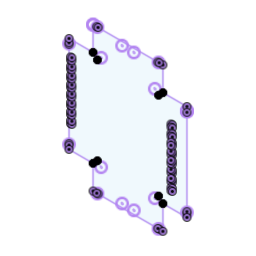
pencil case clasp 2 v8 (Autodesk Fusion 360 design; units mm, degrees)
Autodesk Fusion 360 part; units mm, degrees
sketch "end" plane through (0, 0, 0) normal (0, 1, 0) x (1, 0, 0)
  line L0 (0, 0) -> (10, 0)
  line L1 (10, 0) -> (10, 6)
  line L2 (10, 6) -> (0, 6)
  line L3 (0, 6) -> (0, 0)
  line L4 (0, 0) -> (-10, 0)
  line L5 (-10, 0) -> (-10, 6)
  line L6 (-10, 6) -> (0, 6)
  line L7 (0, 6) -> (0, 0)
  line L8 (0, 3) -> (10, 3) construction
  line L9 (0, 1.2) -> (2, 3)
  line L10 (2, 3) -> (0, 4.8)
  dimension "d1" = 10
  dimension "d2" = 6
  dimension "d3" = 10
  dimension "d4" = 6
  dimension "d5" = 1.2
  dimension "d6" = 1.2
  dimension "d99" = 2
  constraint horizontal L0
  constraint vertical L1
  constraint horizontal L2
  constraint vertical L3
  constraint coincident L0.start L3.end
  constraint horizontal L4
  constraint vertical L5
  constraint horizontal L6
  constraint vertical L7
  constraint midpoint L7 L8.start
  constraint midpoint L1 L8.end
  constraint coincident L3 L9.start
  constraint coincident L3 L10.end
  constraint coincident L8 L9.end
  measures "d1" distance of L0.start L0.end
  measures "d2" distance of L0.start L2.end
  measures "d3" distance of L0.start L4.end
  measures "d4" distance of L0.start L2.end
  measures "d5" distance of L0 L9.start
  measures "d6" distance of L2 L10.end
  measures "d99" distance of L7 L9.end
extrude "Extrude1" add sketch "end" along normal blind 80 contours L0 L1 L2 L3 L7 L9 L10 makes body 1
extrude "Extrude2" add sketch "end" along normal blind 80 separate body contours L3 L4 L5 L6 L7 | L3 L7 L9 L10 makes body 2
sketch "latch" plane through (0, 0, -6) normal (0, 0, -1) x (-1, 0, 0)
  line L0 (-10, 0) -> (0, 0)
  line L1 (0, 0) -> (0, 80)
  line L2 (0, 80) -> (-10, 80)
  line L3 (-10, 80) -> (-10, 0)
  line L4 (0, 0) -> (10, 0)
  line L5 (10, 0) -> (10, 80)
  line L6 (10, 80) -> (0, 80)
  line L7 (0, 80) -> (0, 0)
  line L8 (-10, 0) -> (0, 0)
  line L9 (5, 80) -> (5, 0) construction
  line L10 (10, 66) -> (5, 66)
  line L11 (5, 74) -> (0, 74)
  line L12 (5, 66) -> (5, 74)
  line L13 (5, 66) -> (4.5, 66)
  line L14 (4.5, 66) -> (4.5, 74)
  line L15 (10, 6) -> (-10, 6)
  line L16 (-10, 6) -> (-10, 12)
  line L17 (-10, 12) -> (10, 12)
  line L18 (10, 12) -> (10, 6)
  dimension "d100" = 6
  dimension "d101" = 8
  dimension "d102" = 0.5
  dimension "d116" = 20
  dimension "d117" = 6
  dimension "d118" = 6
  constraint midpoint L6 L9.start
  constraint midpoint L4 L9.end
  constraint coincident L5 L10.start
  constraint coincident L9 L10.end
  constraint perpendicular L9 L10
  constraint coincident L9 L11.start
  constraint coincident L1 L11.end
  constraint perpendicular L1 L11
  constraint perpendicular L9 L13
  constraint coincident L11 L14.end
  constraint perpendicular L11 L14
  constraint horizontal L15
  constraint vertical L16
  constraint horizontal L17
  constraint vertical L18
  constraint coincident L5 L15.start
  measures "d100" distance of L6 L11
  measures "d101" distance of L10 L11
  measures "d102" distance of L10.end L13.end
  measures "d116" distance of L15.start L15.end
  measures "d117" distance of L15.start L17.end
  measures "d118" distance of L4 L15
extrude "Extrude3" cut sketch "latch" against normal blind 6 contours L1 L5 L6 L7 L10 L11 L12 | L11 L12 L13 L14 bodies 2
extrude "Extrude4" add sketch "latch" against normal blind 6 contours L1 L5 L6 L7 L10 L11 L12 bodies 1
extrude "Extrude5" cut 1 faces at (0, 76, -3.6) along direction (1, 0, 0) blind 5 on bodies 2 bodies 2
extrude "Extrude6" add 1 faces at (0, 76, -3.6) along direction (1, 0, 0) blind 4 on bodies 1 bodies 1
chamfer "Chamfer5" distance 2 angle 45 2 edges at (-5, 66, -3) (-4.5, 74, -3) on bodies 1 2
fillet "Fillet8" radius 2 1 edges at (-10, 66, -3) on bodies 1
fillet "Fillet9" radius 2 1 edges at (-10, 66, -3) on bodies 2
fillet "Fillet10" radius 3 2 edges at (-10, 80, -3) (10, 80, -3) on bodies 1
extrude "Extrude16" add sketch "latch" along normal blind 6 contours L1 L3 L7 L15 L16 L17 | L1 L5 L7 L15 L17 L18 bodies 2
fillet "Fillet11" radius 3 4 edges at (10, 12, -9) (10, 6, -9) (-10, 6, -9) (-10, 12, -9) on bodies 2
fillet "Fillet12" radius 2 4 edges at (-10, 9, -12) (0, 12, -12) (10, 9, -12) (0, 6, -12) on bodies 2
sketch "detent" plane through (0, 0, 0) normal (0, 0, 1) x (1, 0, 0)
  arc A0 (-8, 66) -> (-10, 64) centre (-8, 64) ccw
  line L0 (-10, 64) -> (-10, 0)
  line L1 (-10, 0) -> (0, 0)
  line L2 (0, 0) -> (0, 74)
  line L3 (0, 74) -> (-2.5, 74)
  line L4 (-2.5, 74) -> (-4.5, 72)
  line L5 (-4.5, 72) -> (-4.5, 66)
  line L6 (-4.5, 66) -> (-8, 66)
  line L7 (2, 74) -> (0, 74)
  line L8 (0, 74) -> (0, 0)
  line L9 (0, 0) -> (2, 0)
  line L10 (2, 0) -> (2, 74)
  arc A1 (7, 6) -> (7, 12) centre (7, 9) ccw
  line L11 (7, 12) -> (0, 12)
  line L12 (0, 12) -> (0, 6)
  line L13 (0, 6) -> (7, 6)
  circle A2 centre (2, 17) radius 2
  dimension "d133" = 4
  dimension "d134" = 5
  constraint coincident L10 A2.centre
  measures "d133" diameter of A2
  measures "d134" distance of L11 A2.centre
extrude "Extrude17" add sketch "detent" against normal blind 6 contours L10 A2 | L10 A2 bodies 1
extrude "Extrude18" cut sketch "detent" against normal blind 6 contours L10 A2 | L10 A2 bodies 2
copy_body "CopyPasteBodies1" bodies 2 makes body 3
move_body "Move1" bodies 3 to x (-1, 0, 0) y (0, -1, 0) z (0, 0, 1) at (0, 0, 0)
combine "Combine1" operation add target body 1 tool bodies 3
extrude "Extrude9" cut 1 faces at (0.6667, 0, -3) along direction (0, -1, 0) blind 10 on bodies 1 bodies 1
sketch "pins" plane through (0, 0, 0) normal (0, 0, 1) x (1, 0, 0)
  line L0 (10, -64) -> (10, 77)
  line L1 (7, 80) -> (-7, 80)
  line L2 (0, 74) -> (0, -74)
  line L3 (0, 0) -> (18.7462, 0) construction
  line L4 (3.5, 3) -> (6.5, 3)
  line L5 (6.5, 3) -> (6.5, -3)
  line L6 (6.5, -3) -> (3.5, -3)
  line L7 (3.5, -3) -> (3.5, 3)
  line L8 (3.5, 3) -> (6.5, -3) construction
  line L9 (6.5, 3) -> (3.5, -3) construction
  line L10 (6.5, -75) -> (3.5, -75)
  line L11 (3.5, -75) -> (3.5, -69)
  line L12 (3.5, -69) -> (6.5, -69)
  line L13 (6.5, -69) -> (6.5, -75)
  line L14 (6.5, -57) -> (3.5, -57)
  line L15 (3.5, -57) -> (3.5, -51)
  line L16 (3.5, -51) -> (6.5, -51)
  line L17 (6.5, -51) -> (6.5, -57)
  line L18 (6.5, -39) -> (3.5, -39)
  line L19 (3.5, -39) -> (3.5, -33)
  line L20 (3.5, -33) -> (6.5, -33)
  line L21 (6.5, -33) -> (6.5, -39)
  line L22 (6.5, -21) -> (3.5, -21)
  line L23 (3.5, -21) -> (3.5, -15)
  line L24 (3.5, -15) -> (6.5, -15)
  line L25 (6.5, -15) -> (6.5, -21)
  line L26 (6.5, 15) -> (3.5, 15)
  line L27 (3.5, 15) -> (3.5, 21)
  line L28 (3.5, 21) -> (6.5, 21)
  line L29 (6.5, 21) -> (6.5, 15)
  line L30 (6.5, 33) -> (3.5, 33)
  line L31 (3.5, 33) -> (3.5, 39)
  line L32 (3.5, 39) -> (6.5, 39)
  line L33 (6.5, 39) -> (6.5, 33)
  line L34 (6.5, 51) -> (3.5, 51)
  line L35 (3.5, 51) -> (3.5, 57)
  line L36 (3.5, 57) -> (6.5, 57)
  line L37 (6.5, 57) -> (6.5, 51)
  line L38 (6.5, 69) -> (3.5, 69)
  line L39 (3.5, 69) -> (3.5, 75)
  line L40 (3.5, 75) -> (6.5, 75)
  line L41 (6.5, 75) -> (6.5, 69)
  line L42 (9, 80) -> (7, 80)
  line L43 (3.4, -68.9) -> (6.6, -68.9)
  line L44 (6.6, -68.9) -> (6.6, -75.1)
  line L45 (6.6, -75.1) -> (3.4, -75.1)
  line L46 (3.4, -75.1) -> (3.4, -68.9)
  line L47 (3.4, -50.9) -> (6.6, -50.9)
  line L48 (6.6, -50.9) -> (6.6, -57.1)
  line L49 (6.6, -57.1) -> (3.4, -57.1)
  line L50 (3.4, -57.1) -> (3.4, -50.9)
  line L51 (3.4, -32.9) -> (6.6, -32.9)
  line L52 (6.6, -32.9) -> (6.6, -39.1)
  line L53 (6.6, -39.1) -> (3.4, -39.1)
  line L54 (3.4, -39.1) -> (3.4, -32.9)
  line L55 (3.4, -14.9) -> (6.6, -14.9)
  line L56 (6.6, -14.9) -> (6.6, -21.1)
  line L57 (6.6, -21.1) -> (3.4, -21.1)
  line L58 (3.4, -21.1) -> (3.4, -14.9)
  line L59 (3.4, 3.1) -> (6.6, 3.1)
  line L60 (6.6, 3.1) -> (6.6, -3.1)
  line L61 (6.6, -3.1) -> (3.4, -3.1)
  line L62 (3.4, -3.1) -> (3.4, 3.1)
  line L63 (3.4, 21.1) -> (6.6, 21.1)
  line L64 (6.6, 21.1) -> (6.6, 14.9)
  line L65 (6.6, 14.9) -> (3.4, 14.9)
  line L66 (3.4, 14.9) -> (3.4, 21.1)
  line L67 (3.4, 39.1) -> (6.6, 39.1)
  line L68 (6.6, 39.1) -> (6.6, 32.9)
  line L69 (6.6, 32.9) -> (3.4, 32.9)
  line L70 (3.4, 32.9) -> (3.4, 39.1)
  line L71 (3.4, 57.1) -> (6.6, 57.1)
  line L72 (6.6, 57.1) -> (6.6, 50.9)
  line L73 (6.6, 50.9) -> (3.4, 50.9)
  line L74 (3.4, 50.9) -> (3.4, 57.1)
  line L75 (3.4, 75.1) -> (6.6, 75.1)
  line L76 (6.6, 75.1) -> (6.6, 68.9)
  line L77 (6.6, 68.9) -> (3.4, 68.9)
  line L78 (3.4, 68.9) -> (3.4, 75.1)
  arc A0 (10, 77) -> (7, 80) centre (7, 77) ccw
  arc A1 (-7, 80) -> (-10, 77) centre (-7, 77) ccw
  line L79 (-10, 77) -> (-10, 68)
  arc A2 (-10, 68) -> (-8, 66) centre (-8, 68) ccw
  line L80 (-5, 74) -> (0, 74)
  line L81 (0, -74) -> (2.5, -74)
  line L82 (4.5, -72) -> (4.5, -66)
  line L83 (4.5, -66) -> (8, -66)
  arc A3 (8, -66) -> (10, -64) centre (8, -64) ccw
  line L84 (10, -64) -> (0, -64)
  line L85 (0, 74) -> (0, 80)
  line L86 (-7, 66) -> (-5, 68)
  line L87 (-5, 68) -> (-5, 74)
  line L88 (2.5, -74) -> (4.5, -72)
  line L89 (-8, 66) -> (-7, 66)
  point P0 (5, 0)
  dimension "d56" = 3
  dimension "d57" = 6
  dimension "d60" = 0
  dimension "d61" = 18
  dimension "d65" = -0.1
  dimension "d66" = -0.1
  dimension "d67" = -0.1
  dimension "d68" = -0.1
  dimension "d69" = -0.1
  dimension "d70" = -0.1
  dimension "d71" = -0.1
  dimension "d72" = -0.1
  dimension "d73" = -0.1
  dimension "d125" = 5
  constraint coincident L3.start origin
  constraint perpendicular L2 L3
  constraint horizontal L4
  constraint perpendicular L4 L5
  constraint parallel L4 L6
  constraint parallel L5 L7
  constraint coincident L8 P0
  constraint coincident L9 P0
  constraint coincident L3 P0
  constraint coincident L1.start L42.end
  constraint coincident L0.start A3.end
  constraint coincident L2 L84.end
  constraint perpendicular L2 L84
  constraint coincident L2.start L80.end
  constraint midpoint L1 L85.end
  measures "d56" distance of L5.end L6.end
  measures "d57" distance of L4.end L5.end
  measures "d125" distance of L0 P0
extrude "Extrude13" add sketch "pins" along normal blind 2 separate body contours L0 L1 L2 A0 L84 L85 makes body 4
extrude "Extrude14" add sketch "pins" along normal blind 3.5 contours L4 L5 L6 L7 | L14 L15 L16 L17 | L18 L19 L20 L21 | L22 L23 L24 L25 | L26 L27 L28 L29 | L30 L31 L32 L33 | L34 L35 L36 L37 | L38 L39 L40 L41 bodies 1
chamfer "Chamfer4" distance 1 angle 45 32 edges at (5, -57.1, 2) (3.4, -54, 2) (5, -50.9, 2) (6.6, -54, 2) (5, -39.1, 2) (3.4, -36, 2) (5, -32.9, 2) (6.6, -36, 2) (5, -21.1, 2) (3.4, -18, 2) (5, -14.9, 2) (6.6, -18, 2) (5, -3.1, 2) (3.4, 0, 2) (6.6, 0, 2) (5, 3.1, 2) (5, 14.9, 2) (3.4, 18, 2) (6.6, 18, 2) (5, 21.1, 2) (5, 32.9, 2) (3.4, 36, 2) (6.6, 36, 2) (5, 39.1, 2) (5, 50.9, 2) (6.6, 54, 2) (3.4, 54, 2) (5, 57.1, 2) (5, 68.9, 2) (6.6, 72, 2) (3.4, 72, 2) (5, 75.1, 2) tangent chain off on bodies 4
fillet "Fillet4" radius 1 1 faces at (5.8667, -62.0333, 2) on bodies 4
fillet "Fillet5" radius 1 10 edges at (0, 80, -6) (-9.1213, 79.1213, -6) (-10, 72.5, -6) (-9.4142, 66.5858, -6) (-7.5, 66, -6) (9.1213, 79.1213, -6) (10, 34, -6) (10, -36.5, -6) (9.4142, -65.4142, -6) (6.25, -66, -6) on bodies 1
fillet "Fillet6" radius 1 2 edges at (-2, -12.5, -3) (-2, -46.5, -3) on bodies 1
sketch "fabric layout" plane through (0, 0, 0) normal (0, 0, 1) x (1, 0, 0)
  line L0 (3.4, 75.1) -> (6.6, 75.1)
  line L1 (3.4, 57.1) -> (6.6, 57.1)
  line L2 (3.4, 39.1) -> (6.6, 39.1)
  line L3 (3.4, 21.1) -> (6.6, 21.1)
  line L4 (3.4, 3.1) -> (6.6, 3.1)
  line L5 (3.4, -14.9) -> (6.6, -14.9)
  line L6 (3.4, -32.9) -> (6.6, -32.9)
  line L7 (3.4, -50.9) -> (6.6, -50.9)
  line L8 (3.4, -39.1) -> (3.4, -32.9)
  line L9 (6.6, -39.1) -> (3.4, -39.1)
  line L10 (3.4, 68.9) -> (3.4, 75.1)
  line L11 (6.6, 68.9) -> (3.4, 68.9)
  line L12 (3.4, -57.1) -> (3.4, -50.9)
  line L13 (6.6, -57.1) -> (3.4, -57.1)
  line L14 (3.4, 50.9) -> (3.4, 57.1)
  line L15 (6.6, 50.9) -> (3.4, 50.9)
  line L16 (3.4, 32.9) -> (3.4, 39.1)
  line L17 (6.6, 32.9) -> (3.4, 32.9)
  line L18 (3.4, -3.1) -> (3.4, 3.1)
  line L19 (6.6, -3.1) -> (3.4, -3.1)
  line L20 (3.4, 14.9) -> (3.4, 21.1)
  line L21 (6.6, 14.9) -> (3.4, 14.9)
  line L22 (3.4, -21.1) -> (3.4, -14.9)
  line L23 (6.6, -21.1) -> (3.4, -21.1)
  line L24 (0, -64) -> (0, 80)
  line L25 (7, 80) -> (0, 80)
  line L26 (0, 0) -> (0, 100) construction
  line L27 (0, 100) -> (30, 100) construction
  line L28 (30, 100) -> (90, 100) construction
  line L29 (90, 100) -> (120, 100) construction
  line L30 (0, 0) -> (0, 165)
  line L31 (0, 165) -> (120, 165)
  circle A0 centre (0, 100) radius 1.5
  line L32 (120, 165) -> (120, 2.0082) construction
  line L33 (236.6, -50.9) -> (233.4, -50.9)
  line L34 (236.6, -57.1) -> (236.6, -50.9)
  line L35 (150, 100) -> (120, 100) construction
  line L36 (233.4, -21.1) -> (236.6, -21.1)
  line L37 (236.6, -14.9) -> (233.4, -14.9)
  line L38 (236.6, -32.9) -> (233.4, -32.9)
  line L39 (233.4, -3.1) -> (236.6, -3.1)
  line L40 (233.4, -57.1) -> (236.6, -57.1)
  line L41 (233.4, -50.9) -> (233.4, -57.1)
  line L42 (240, 165) -> (120, 165)
  line L43 (236.6, -21.1) -> (236.6, -14.9)
  line L44 (236.6, 3.1) -> (233.4, 3.1)
  line L45 (236.6, -3.1) -> (236.6, 3.1)
  line L46 (233.4, -39.1) -> (236.6, -39.1)
  line L47 (233.4, 3.1) -> (233.4, -3.1)
  line L48 (233.4, 21.1) -> (233.4, 14.9)
  line L49 (236.6, 21.1) -> (233.4, 21.1)
  line L50 (233.4, 32.9) -> (236.6, 32.9)
  line L51 (236.6, 57.1) -> (233.4, 57.1)
  line L52 (233.4, 50.9) -> (236.6, 50.9)
  line L53 (233.4, 57.1) -> (233.4, 50.9)
  line L54 (240, 100) -> (210, 100) construction
  line L55 (210, 100) -> (150, 100) construction
  line L56 (236.6, 50.9) -> (236.6, 57.1)
  line L57 (236.6, 39.1) -> (233.4, 39.1)
  line L58 (240, 0) -> (240, 100) construction
  line L59 (233.4, 39.1) -> (233.4, 32.9)
  line L60 (236.6, -39.1) -> (236.6, -32.9)
  line L61 (236.6, 32.9) -> (236.6, 39.1)
  line L62 (233.4, -32.9) -> (233.4, -39.1)
  line L63 (233.4, -14.9) -> (233.4, -21.1)
  line L64 (236.6, 14.9) -> (236.6, 21.1)
  line L65 (233.4, 14.9) -> (236.6, 14.9)
  line L66 (240, 165) -> (270, 165)
  line L67 (0, 0) -> (393.973, 0) construction
  line L68 (270, 165) -> (270, 0)
  arc A1 (10, 77) -> (7, 80) centre (7, 77) ccw
  line L69 (10, -64) -> (10, 77)
  line L70 (6.6, 75.1) -> (6.6, 68.9)
  line L71 (6.6, 57.1) -> (6.6, 50.9)
  line L72 (6.6, 39.1) -> (6.6, 32.9)
  line L73 (6.6, 21.1) -> (6.6, 14.9)
  line L74 (6.6, 3.1) -> (6.6, -3.1)
  line L75 (6.6, -14.9) -> (6.6, -21.1)
  line L76 (6.6, -32.9) -> (6.6, -39.1)
  line L77 (6.6, -50.9) -> (6.6, -57.1)
  line L78 (10, -64) -> (0, -64)
  line L79 (0, 100) -> (65, 100)
  line L80 (65, 100) -> (65, 165)
  line L81 (270, 100) -> (205, 100)
  line L82 (205, 100) -> (205, 165)
  line L83 (140, 165) -> (205, 100) construction
  line L84 (130, 165) -> (65, 100) construction
  line L85 (130, 165) -> (181.9186, 165) construction
  circle A2 centre (65, 100) radius 1.5
  circle A3 centre (205, 100) radius 1.5
  line L86 (270, 110) -> (268.1505, 110)
  line L87 (268.1505, 110) -> (215, 110)
  line L88 (215, 110) -> (215, 165)
  line L89 (55, 165) -> (55, 110)
  line L90 (55, 110) -> (0, 110)
  line L91 (55, 110) -> (65, 100)
  line L92 (205, 100) -> (215, 110)
  circle A4 centre (121.5147, 156.5147) radius 1.5
  circle A5 centre (73.4853, 108.4853) radius 1.5
  circle A6 centre (196.5147, 108.4853) radius 1.5
  circle A7 centre (148.4853, 156.5147) radius 1.5
  line L93 (0, 0) -> (0, -100) construction
  line L94 (0, 0) -> (0, -165)
  line L95 (55, -110) -> (0, -110)
  line L96 (0, -100) -> (65, -100)
  line L97 (55, -110) -> (65, -100)
  line L98 (65, -100) -> (130, -165)
  line L99 (55, -165) -> (55, -110)
  line L100 (0, -165) -> (120, -165)
  line L101 (130, -165) -> (181.9186, -165) construction
  line L102 (240, -165) -> (120, -165)
  line L103 (205, -100) -> (140, -165)
  line L104 (205, -100) -> (215, -110)
  line L105 (240, -100) -> (210, -100) construction
  line L106 (270, -100) -> (205, -100)
  line L107 (268.1505, -110) -> (215, -110)
  line L108 (215, -110) -> (215, -165)
  line L109 (270, -165) -> (270, 0)
  line L110 (240, -165) -> (270, -165)
  circle A8 centre (121.5147, -156.5147) radius 1.5
  circle A9 centre (73.4853, -108.4853) radius 1.5
  circle A10 centre (196.5147, -108.4853) radius 1.5
  circle A11 centre (270, 100) radius 1.5
  circle A12 centre (0, -100) radius 1.5
  circle A13 centre (65, -100) radius 1.5
  circle A14 centre (130, -165) radius 1.5
  circle A15 centre (121.5147, -156.5147) radius 1.5
  circle A16 centre (73.4853, -108.4853) radius 1.5
  circle A17 centre (196.5147, -108.4853) radius 1.5
  circle A18 centre (148.4853, -156.5147) radius 1.5
  circle A19 centre (205, -100) radius 1.5
  circle A20 centre (270, -100) radius 1.5
  line L111 (233.4, -68.9) -> (236.6, -68.9)
  line L112 (233.4, -75.1) -> (233.4, -68.9)
  line L113 (236.6, -68.9) -> (236.6, -75.1)
  line L114 (236.6, -75.1) -> (233.4, -75.1)
  line L115 (268.1505, -110) -> (215, -110)
  line L116 (270, -110) -> (268.1505, -110)
  circle A21 centre (65, 165) radius 1.5
  circle A22 centre (205, 165) radius 1.5
  line L117 (65, -100) -> (65, -165)
  line L118 (205, -100) -> (205, -165)
  circle A23 centre (205, -165) radius 1.5
  circle A24 centre (65, -165) radius 1.5
  point P0 (7, 80)
  point P1 (233, 80)
  point P2 (240, 0)
  point P3 (120, 2.0082)
  point P4 (148.4853, -156.5147)
  dimension "d85" = 100
  dimension "d86" = 30
  dimension "d87" = 60
  dimension "d88" = 30
  dimension "d89" = 20
  dimension "d90" = 65
  dimension "d91" = 3
  dimension "d92" = 120
  dimension "d93" = 30
  dimension "d143" = 65
  dimension "d144" = 65
  dimension "d145" = 315
  dimension "d146" = 135
  dimension "d147" = 30
  dimension "d148" = 3
  dimension "d149" = 3
  dimension "d150" = 10
  dimension "d151" = 10
  dimension "d152" = 10
  dimension "d153" = 10
  dimension "d154" = 3
  dimension "d155" = 3
  dimension "d156" = 3
  dimension "d157" = 3
  dimension "d158" = 12
  dimension "d159" = 12
  dimension "d160" = 12
  dimension "d161" = 12
  dimension "d162" = 65
  dimension "d165" = 3
  dimension "d166" = 3
  dimension "d167" = 3
  constraint coincident L26.start L30.start
  constraint perpendicular L4 L26
  constraint perpendicular L24 L27
  constraint parallel L27 L28
  constraint parallel L28 L29
  constraint perpendicular L27 L30
  constraint perpendicular L26 L31
  constraint coincident L26.end L27.start
  constraint perpendicular L31 L32
  constraint symmetric L26.start L32 P2
  constraint symmetric L1.end L32 L51.end
  constraint symmetric L15.start L32 L52.start
  constraint symmetric L1.start L32 L51.start
  constraint symmetric L2.end L32 L57.end
  constraint symmetric L17.start L32 L50.start
  constraint symmetric L2.start L32 L57.start
  constraint symmetric L3.end L32 L48.start
  constraint symmetric L21.start L32 L48.end
  constraint symmetric L3.start L32 L49.start
  constraint symmetric L4.end L32 L44.end
  constraint symmetric L19.start L32 L39.start
  constraint symmetric L4.start L32 L44.start
  constraint symmetric L5.end L32 L37.end
  constraint symmetric L23.start L32 L36.start
  constraint symmetric L5.start L32 L37.start
  constraint symmetric L6.end L32 L38.end
  constraint symmetric L9.start L32 L46.start
  constraint symmetric L6.start L32 L38.start
  constraint symmetric L7.end L32 L33.end
  constraint symmetric L13.start L32 L40.start
  constraint symmetric L7.start L32 L33.start
  constraint symmetric L8.start L32 L46.end
  constraint symmetric L12.start L32 L34.start
  constraint symmetric L14.start L32 L52.end
  constraint symmetric L16.start L32 L50.end
  constraint symmetric L18.start L32 L39.end
  constraint symmetric L20.start L32 L64.start
  constraint symmetric L22.start L32 L36.end
  constraint symmetric L26.end L32 L54.start
  constraint symmetric L27.end L32 L54.end
  constraint symmetric L28.end L32 L35.start
  constraint symmetric L29.end L32 L35.end
  constraint symmetric P0 L32 P1
  constraint symmetric L30.end L32 L42.start
  constraint symmetric L31.end L32 L42.end
  constraint symmetric P3 L32 L32.end
  constraint coincident L67 L68.end
  constraint perpendicular L67 L68
  constraint parallel L28 L79
  constraint coincident L31 L84.start
  constraint perpendicular L31 L80
  constraint coincident L68 L81.start
  constraint perpendicular L58 L81
  constraint coincident L42 L83.start
  constraint perpendicular L42 L82
  constraint coincident L35 L81.end
  constraint horizontal L85
  constraint coincident L35 L79.end
  constraint coincident L79.end L80.start
  constraint coincident L81.end L82.start
  constraint coincident L68 L86.start
  constraint perpendicular L68 L86
  constraint parallel L86 L87
  constraint coincident L42 L88.end
  constraint perpendicular L42 L88
  constraint coincident L31 L89.start
  constraint perpendicular L31 L89
  constraint coincident L30 L90.end
  constraint perpendicular L30 L90
  constraint coincident L84 A4.centre
  constraint coincident L84 A5.centre
  constraint coincident L83 A6.centre
  constraint coincident L83 A7.centre
  constraint coincident L67 L26.start
  constraint symmetric L26.start L67 L30.start
  constraint symmetric L26.end L67 L93.end
  constraint symmetric L30.end L67 L94.end
  constraint symmetric L31.end L67 L100.end
  constraint symmetric L54.end L67 L105.end
  constraint symmetric L42.start L67 L102.start
  constraint symmetric L54.start L67 L105.start
  constraint symmetric L66.end L67 L109.start
  constraint symmetric L67 L68.end L109.end
  constraint symmetric L67 L26.end L93.end
  constraint symmetric L67 L79.end L96.end
  constraint symmetric L67 L84.start L98.end
  constraint symmetric L67 L81.start L106.start
  constraint symmetric L67 L81.end L103.start
  constraint symmetric L67 L83.start L103.end
  constraint symmetric L67 L85.end L101.end
  constraint symmetric L67 L86.end L107.start
  constraint symmetric L67 L87.end L104.end
  constraint symmetric L67 L88.end L108.end
  constraint symmetric L67 L89.start L99.start
  constraint symmetric L67 L89.end L95.start
  constraint symmetric L67 L90.end L95.end
  constraint symmetric L67 A4 A8
  constraint symmetric L67 A5 A9
  constraint symmetric L67 A6 A10
  constraint symmetric L67 A7.centre P4
  constraint symmetric L67 L26.start L30.start
  constraint coincident L81.start A11.centre
  constraint symmetric A0 L67 A12
  constraint symmetric L67 A2 A13
  constraint symmetric L67 A3 A19
  constraint symmetric L67 A4 A15
  constraint symmetric L67 A5 A16
  constraint symmetric L67 A6 A17
  constraint symmetric L67 A7 A18
  constraint symmetric L67 A11 A20
  constraint symmetric L67 L86.start L116.start
  constraint coincident L84 L79.end
  constraint coincident L80.end A21.centre
  constraint coincident L82.end A22.centre
  constraint coincident L83 L81.end
  constraint symmetric L67 L80.end L117.end
  constraint symmetric L67 A21 A24
  constraint symmetric L67 L82.end L118.end
  constraint symmetric L67 A22 A23
  measures "d85" distance of L26.start L26.end
  measures "d86" distance of L26.end L27.end
  measures "d87" distance of L27.end L28.end
  measures "d88" distance of L28.end L29.end
  measures "d89" distance of L27 P0
  measures "d90" distance of L27 L31
  measures "d91" diameter of A0
  measures "d92" distance of L26 L32
  measures "d93" distance of L42.start L66.end
  measures "d143" distance of L26.end L79.end
  measures "d144" distance of L81.start L81.end
  measures "d146" angle of L84 L85
  measures "d147" distance of L58 L68
  measures "d148" diameter of A2
  measures "d149" diameter of A3
  measures "d150" distance of L80 L89
  measures "d151" distance of L28 L90
  measures "d152" distance of L82 L88
  measures "d153" distance of L81 L87
  measures "d154" diameter of A4
  measures "d155" diameter of A5
  measures "d156" diameter of A6
  measures "d157" diameter of A7
  measures "d158" distance of L83.start A7.centre
  measures "d159" distance of L84.start A4.centre
  measures "d160" distance of L81.end A6.centre
  measures "d161" distance of L79.end A5.centre
  measures "d162" distance of L66 L81
  measures "d165" diameter of A11
  measures "d166" diameter of A21
  measures "d167" diameter of A22
extrude "Extrude15" add sketch "fabric layout" along normal blind 3 separate body contours L24 L25 L30 A1 L69 L78 L94 | L25 L30 L31 A0 L42 L68 A1 L69 L78 L79 L80 L81 L82 A2 A3 L94 L96 L98 L102 L103 L106 L109 A8 A9 A10 A11 A12 A13 A14 A15 A16 A17 A18 A19 A20 A21 A22 | L94 L95 L96 L97 A12 A13 | L30 A0 L79 A2 L90 L91 | L97 L99 L100 A13 L117 A24 | L98 L100 L102 A8 A9 A13 A14 A15 A16 L117 A24 | L31 L80 A2 L89 L91 A21 | L98 L102 A14 | L98 L102 A14 | L102 L103 A10 A17 A18 A19 L118 A23 | L42 L82 A3 L88 L92 A22 | L102 L104 L108 A19 L118 A23 | L68 L81 A3 L86 L87 L92 A11 | L104 L106 L107 L109 A19 A20 L115 L116 makes body 5
sketch "pencil case 2 fabric" plane through (0, 0, 0) normal (0, 0, 1) x (1, 0, 0)
  circle A0 centre (148.4853, 156.5147) radius 1.5
  line L0 (236.6, -3.1) -> (233.4, -3.1)
  line L1 (236.6, 3.1) -> (236.6, -3.1)
  line L2 (233.4, 3.1) -> (236.6, 3.1)
  line L3 (233.4, -3.1) -> (233.4, 3.1)
  line L4 (233.4, 57.1) -> (236.6, 57.1)
  line L5 (233.4, 50.9) -> (233.4, 57.1)
  line L6 (236.6, 50.9) -> (233.4, 50.9)
  line L7 (236.6, 57.1) -> (236.6, 50.9)
  line L8 (233.4, 39.1) -> (236.6, 39.1)
  line L9 (233.4, 32.9) -> (233.4, 39.1)
  line L10 (236.6, 32.9) -> (233.4, 32.9)
  line L11 (236.6, 39.1) -> (236.6, 32.9)
  line L12 (236.6, -39.1) -> (233.4, -39.1)
  line L13 (236.6, -32.9) -> (236.6, -39.1)
  line L14 (233.4, -32.9) -> (236.6, -32.9)
  line L15 (233.4, -39.1) -> (233.4, -32.9)
  line L16 (236.6, -21.1) -> (233.4, -21.1)
  line L17 (236.6, -14.9) -> (236.6, -21.1)
  line L18 (233.4, -14.9) -> (236.6, -14.9)
  line L19 (233.4, -21.1) -> (233.4, -14.9)
  circle A1 centre (196.5147, 108.4853) radius 1.5
  line L20 (236.6, 21.1) -> (236.6, 14.9)
  line L21 (233.4, 21.1) -> (236.6, 21.1)
  line L22 (233.4, 14.9) -> (233.4, 21.1)
  line L23 (236.6, 14.9) -> (233.4, 14.9)
  circle A2 centre (73.4853, 108.4853) radius 1.5
  circle A3 centre (121.5147, 156.5147) radius 1.5
  line L24 (236.6, -57.1) -> (233.4, -57.1)
  line L25 (236.6, -50.9) -> (236.6, -57.1)
  line L26 (233.4, -50.9) -> (236.6, -50.9)
  line L27 (233.4, -57.1) -> (233.4, -50.9)
  line L28 (233.4, -68.9) -> (236.6, -68.9)
  line L29 (233.4, -75.1) -> (233.4, -68.9)
  line L30 (236.6, -75.1) -> (233.4, -75.1)
  line L31 (236.6, -68.9) -> (236.6, -75.1)
  circle A4 centre (121.5147, -156.5147) radius 1.5
  circle A5 centre (73.4853, -108.4853) radius 1.5
  circle A6 centre (196.5147, -108.4853) radius 1.5
  circle A7 centre (148.4853, -156.5147) radius 1.5
  arc A8 (270, 101.5) -> (270, 98.5) centre (270, 100) ccw
  line L32 (270, 110) -> (270, 101.5)
  arc A9 (270, -98.5) -> (270, -101.5) centre (270, -100) ccw
  arc A10 (0, -101.5) -> (0, -98.5) centre (0, -100) ccw
  arc A11 (0, 98.5) -> (0, 101.5) centre (0, 100) ccw
  line L33 (3.4, -57.1) -> (3.4, -50.9)
  line L34 (6.6, -57.1) -> (3.4, -57.1)
  line L35 (6.6, -50.9) -> (6.6, -57.1)
  line L36 (3.4, -50.9) -> (6.6, -50.9)
  line L37 (3.4, -39.1) -> (3.4, -32.9)
  line L38 (6.6, -39.1) -> (3.4, -39.1)
  line L39 (6.6, -32.9) -> (6.6, -39.1)
  line L40 (3.4, -32.9) -> (6.6, -32.9)
  line L41 (3.4, -21.1) -> (3.4, -14.9)
  line L42 (6.6, -21.1) -> (3.4, -21.1)
  line L43 (6.6, -14.9) -> (6.6, -21.1)
  line L44 (3.4, -14.9) -> (6.6, -14.9)
  line L45 (3.4, -3.1) -> (3.4, 3.1)
  line L46 (6.6, -3.1) -> (3.4, -3.1)
  line L47 (6.6, 3.1) -> (6.6, -3.1)
  line L48 (3.4, 3.1) -> (6.6, 3.1)
  line L49 (3.4, 14.9) -> (3.4, 21.1)
  line L50 (6.6, 14.9) -> (3.4, 14.9)
  line L51 (6.6, 21.1) -> (6.6, 14.9)
  line L52 (3.4, 21.1) -> (6.6, 21.1)
  line L53 (3.4, 32.9) -> (3.4, 39.1)
  line L54 (6.6, 32.9) -> (3.4, 32.9)
  line L55 (6.6, 39.1) -> (6.6, 32.9)
  line L56 (3.4, 39.1) -> (6.6, 39.1)
  line L57 (3.4, 50.9) -> (3.4, 57.1)
  line L58 (6.6, 50.9) -> (3.4, 50.9)
  line L59 (6.6, 57.1) -> (6.6, 50.9)
  line L60 (3.4, 57.1) -> (6.6, 57.1)
  line L61 (3.4, 68.9) -> (3.4, 75.1)
  line L62 (6.6, 68.9) -> (3.4, 68.9)
  line L63 (6.6, 75.1) -> (6.6, 68.9)
  line L64 (3.4, 75.1) -> (6.6, 75.1)
  line L65 (0, -98.5) -> (0, 98.5)
  circle A12 centre (205, 100) radius 1.5
  circle A13 centre (205, -100) radius 1.5
  circle A14 centre (65, -100) radius 1.5
  circle A15 centre (65, 100) radius 1.5
  line L66 (270, -110) -> (270, -101.5)
  line L67 (66.5, -165) -> (203.5, -165)
  line L68 (55, -165) -> (55, -110)
  line L69 (55, -110) -> (0, -110)
  line L70 (0, -101.5) -> (0, -110)
  line L71 (0, 101.5) -> (0, 110)
  line L72 (55, 110) -> (0, 110)
  line L73 (55, 165) -> (55, 110)
  line L74 (215, 110) -> (215, 165)
  line L75 (270, 110) -> (215, 110)
  line L76 (270, -110) -> (215, -110)
  line L77 (215, -110) -> (215, -165)
  line L78 (270, -98.5) -> (270, 98.5)
  line L79 (215, -165) -> (206.5, -165)
  line L80 (55, 165) -> (63.5, 165)
  arc A16 (206.5, -165) -> (203.5, -165) centre (205, -165) ccw
  arc A17 (66.5, -165) -> (63.5, -165) centre (65, -165) ccw
  line L81 (55, -165) -> (63.5, -165)
  arc A18 (63.5, 165) -> (66.5, 165) centre (65, 165) ccw
  line L82 (203.5, 165) -> (66.5, 165)
  arc A19 (203.5, 165) -> (206.5, 165) centre (205, 165) ccw
  line L83 (215, 165) -> (206.5, 165)
  line L84 (55, -110) -> (65, -100)
  line L85 (215, -110) -> (205, -100)
  line L86 (215, 110) -> (205, 100)
  line L87 (55, 110) -> (65, 100)
  constraint coincident L68.end L69.start
  constraint coincident A14.centre L84.end
  constraint coincident L76.end L77.start
  constraint coincident A13.centre L85.end
  constraint coincident L74.start L75.end
  constraint coincident A12.centre L86.end
  constraint coincident L72.start L73.end
  constraint coincident A15.centre L87.end
chamfer "Chamfer7" distance 1 distance2 1 3 edges at (-0.5871, -74, -4.2716) (-1.5052, -74, -3) (-0.5871, -74, -1.7284) measured on face at (-0.7827, -55.6072, -4.0955) measured on face at (-1.4613, -37.2824, -3.2928) measured on face at (-0.7827, -55.6072, -1.9045) on bodies 1
move_face "OffsetFaces1" offset -0.75 1 faces at (-4.6671, -10, -6) on bodies 1
move_face "OffsetFaces2" offset -3 1 faces at (-0.1161, -10, -3) on bodies 1
chamfer "Chamfer8" distance 2 distance2 1 3 edges at (-0.5871, -13, -1.7284) (-1.5052, -13, -3) (-0.5871, -13, -4.2716) measured on face at (-0.683, -13.7822, -1.8147) measured on face at (-1.2258, -13.7182, -2.3067) measured on face at (-0.7089, -13.7654, -4.162) on bodies 1
fillet "Fillet13" radius 2 2 edges at (2.5, -74, -3) (4.5, -72, -3) on bodies 1
fillet "Fillet14" radius 2 1 edges at (-5, 68, -3) on bodies 1
hidden bodies 1 2 4 5
equation "d145 = 360 deg - 45 deg"
named bodies: "pencil case 2 clasp", "pencil case 2 backer", "fabric"
